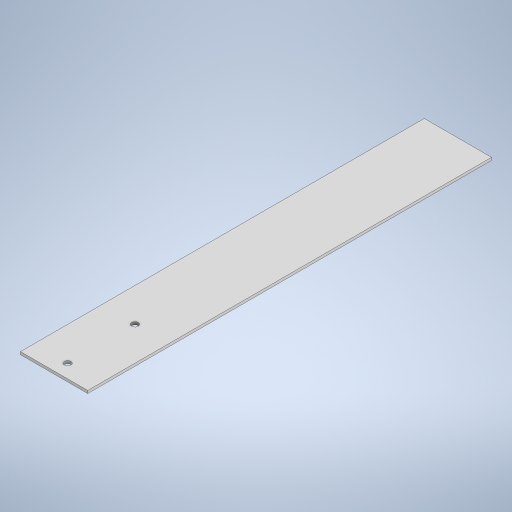
# Autodesk Inventor part: Ldw
Saved by Autodesk Inventor 2023 (Build 270158000, 158)
## iProperties
Created: 2022-11-06
Part Number: Ldw
Material: Generic
Document SubType Name: Modeling
Designer: SAMJ
Density: 1 g/cm^3
Appearance: Default
Author: SAMJ
Autodesk Inventor part; units mm, degrees
ref_plane "YZ Plane" through (0, 0, 0) normal (1, 0, 0) x (0, 1, 0)
ref_plane "XZ Plane" through (0, 0, 0) normal (0, 1, 0) x (-1, 0, 0)
ref_plane "XY Plane" through (0, 0, 0) normal (0, 0, 1) x (1, 0, 0)
sketch "Sketch1" plane through (0, 0, 0) normal (0, 1, 0) x (-1, 0, 0)
  line L0 (-25, 150) -> (25, 150)
  line L1 (25, 150) -> (25, -150)
  line L2 (25, -150) -> (-25, -150)
  line L3 (-25, -150) -> (-25, 150)
  line L4 (-25, 150) -> (25, -150) construction
  line L5 (25, 150) -> (-25, -150) construction
  line L6 (0, 150) -> (0, 140)
  circle A0 centre (0, 140) radius 2.5
  line L7 (0, 140) -> (0, 90)
  circle A1 centre (0, 90) radius 2.5
  point P0 (0, 0)
  dimension "d0" = 50
  dimension "d1" = 300
  dimension "d2" = 10
  dimension "d3" = 5
  dimension "d4" = 50
  dimension "d5" = 5
  constraints: 16 end point, 3 midpoint, 2 centre point, 2 coincident, 2 parallel, 2 vertical, 1 horizontal, 1 perpendicular
  measures "d0" distance of L1.end L2.end
  measures "d1" distance of L0.end L1.end
  measures "d2" distance of L6.start L6.end
  measures "d3" diameter of A0
  measures "d4" distance of L7.start L7.end
  measures "d5" diameter of A1
extrude "Extrusion1" add sketch "Sketch1" along normal blind 2
body "Solid1"
